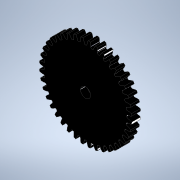
# Autodesk Inventor part: Engranaje
Saved by Autodesk Inventor 2020.3 (Build 243373000, 373)
## iProperties
Created: 2021-02-24
Part Number: Engranaje
Material: PET Plastic
Document SubType Name: Modeling
Designer: juanp
Density: 1.541 g/cm^3
Appearance: Polycarbonate - Clear
Author: juanp
Autodesk Inventor part; units mm, degrees
ref_plane "YZ Plane" through (0, 0, 0) normal (1, 0, 0) x (0, 1, 0)
ref_plane "XZ Plane" through (0, 0, 0) normal (0, 1, 0) x (-1, 0, 0)
ref_plane "XY Plane" through (0, 0, 0) normal (0, 0, 1) x (1, 0, 0)
sketch "Sketch1" plane through (0, 0, 0) normal (0, 0, 1) x (1, 0, 0)
  spline S0 degree 3 poles (-1.1768, 20.967) (-1.128, 20.8639) (-1.0547, 20.7094) (-0.9668, 20.4989) (-0.9045, 20.3396) (-0.8467, 20.1786) (-0.7937, 20.0159) (-0.746, 19.8516) (-0.705, 19.6856) (-0.6701, 19.518) (-0.6556, 19.3761) (-0.6413, 19.263) (-0.626, 19.1788) (-0.6032, 19.0962) (-0.573, 19.0161) (-0.5327, 18.9404) (-0.4886, 18.8839) (-0.4476, 18.8443) (-0.4136, 18.8183) (-0.3775, 18.7952) (-0.3386, 18.7771) (-0.2983, 18.7628) (-0.2425, 18.75) (-0.1423, 18.7482) (0, 18.7512) (0.1423, 18.7482) (0.2425, 18.75) (0.2983, 18.7628) (0.3386, 18.7771) (0.3775, 18.7952) (0.4136, 18.8183) (0.4476, 18.8443) (0.4886, 18.8839) (0.5327, 18.9404) (0.573, 19.0161) (0.6032, 19.0962) (0.626, 19.1788) (0.6413, 19.263) (0.6556, 19.3761) (0.6701, 19.518) (0.705, 19.6856) (0.746, 19.8516) (0.7937, 20.0159) (0.8467, 20.1786) (0.9045, 20.3396) (0.9668, 20.4989) (1.0547, 20.7094) (1.128, 20.8639) (1.1768, 20.967) knots 0 0 0 0 0.034206 0.05131 0.068414 0.085518 0.102622 0.119726 0.136829 0.153931 0.17103 0.179582 0.188133 0.196683 0.20523 0.213776 0.222318 0.226595 0.230868 0.235144 0.239418 0.243694 0.247969 0.256512 0.273616 0.29072 0.299263 0.303538 0.307814 0.312088 0.316363 0.320637 0.324913 0.333456 0.342002 0.350549 0.359099 0.36765 0.376201 0.393301 0.410403 0.427506 0.44461 0.461714 0.478818 0.495922 0.513026 0.547232 0.547232 0.547232 0.547232
  circle A0 centre (0, 0) radius 18.75 construction
  circle A1 centre (0, 0) radius 19.363 construction
  circle A2 centre (0, 0) radius 20 construction
  circle A3 centre (0, 0) radius 21
  point P0 (-1.0336, 20.6564)
  point P1 (-0.9674, 20.4986)
  point P2 (-0.9053, 20.3393)
  point P3 (-0.8475, 20.1783)
  point P4 (-0.7946, 20.0157)
  point P5 (-0.7471, 19.8514)
  point P6 (-0.706, 19.6853)
  point P7 (-0.673, 19.5175)
  point P8 (-0.6518, 19.3478)
  point P9 (-0.6405, 19.2631)
  point P10 (-0.6247, 19.179)
  point P11 (-0.602, 19.0966)
  point P12 (-0.5713, 19.0168)
  point P13 (-0.5306, 18.9417)
  point P14 (-0.4779, 18.8745)
  point P15 (-0.447, 18.8449)
  point P16 (-0.4132, 18.8187)
  point P17 (-0.377, 18.796)
  point P18 (-0.3384, 18.7778)
  point P19 (-0.298, 18.7636)
  point P20 (-0.2563, 18.7542)
  point P21 (-0.171, 18.7491)
  point P22 (0, 18.75)
  point P23 (0.171, 18.7491)
  point P24 (0.2563, 18.7542)
  point P25 (0.298, 18.7636)
  point P26 (0.3384, 18.7778)
  point P27 (0.377, 18.796)
  point P28 (0.4132, 18.8187)
  point P29 (0.447, 18.8449)
  point P30 (0.4779, 18.8745)
  point P31 (0.5306, 18.9417)
  point P32 (0.5713, 19.0168)
  point P33 (0.602, 19.0966)
  point P34 (0.6247, 19.179)
  point P35 (0.6405, 19.2631)
  point P36 (0.6518, 19.3478)
  point P37 (0.673, 19.5175)
  point P38 (0.706, 19.6853)
  point P39 (0.7471, 19.8514)
  point P40 (0.7946, 20.0157)
  point P41 (0.8475, 20.1783)
  point P42 (0.9053, 20.3393)
  point P43 (0.9674, 20.4986)
  point P44 (1.0336, 20.6564)
  constraints: 4 centre point, 2 point on circle, 99 other
extrude "Extrusion1" add sketch "Sketch1" against normal mid plane 4
extrude "Extrusion2" cut sketch "Sketch1" against normal mid plane 10 contours A3 S0 picked at (-0.0926, 20.2811)
pattern_circular "Circular Pattern1" count 40 over 360 about axis through (0, 0, 0) along (0, 0, -1) of "Extrusion2"
sketch "Sketch2" plane through (0, 0, 2) normal (0, 0, 1) x (1, 0, 0)
  circle A0 centre (0, 0) radius 2.3
  circle A1 centre (0, 0) radius 1.25
  dimension "d7" = 4.6
  dimension "d10" = 2.5
  constraints: 2 centre point, 2 coincident
  measures "d7" diameter of A0
  measures "d10" diameter of A1
extrude "Extrusion3" cut sketch "Sketch2" against normal blind 3 contours A0 | A1
extrude "Extrusion4" cut sketch "Sketch2" against normal blind 10 contours A1
equation "\"Module\" = 1"
equation "\"PressureAngle\" = 14.5deg"
equation "\"UnitProfileClearance\" = 0.25"
equation "\"UnitRoundRadius\" = 0.3335"
equation "\"HeadDiameter\" = 42"
equation "\"RootDiameter\" = 37.5"
equation "\"BaseDiameter\" = 38.72591"
equation "\"FaceWidth\" = 5"
equation "\"HelixAngle\" = 0"
equation "\"UnitCorrection\" = 0"
equation "\"UnitAddendumModification\" = 0"
equation "\"CircularPitch\" = 3.141593"
equation "\"UnitBacklashShift\" = 0"
equation "\"TotalToolShift\" = 0"
equation "\"IsInternal\" = 0"
body "Solid1"
